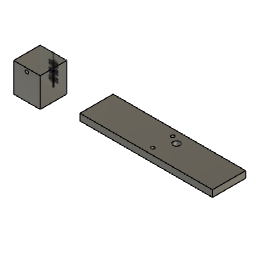
Phantom3 (Autodesk Fusion 360 design; units mm, degrees)
Autodesk Fusion 360 part; units mm, degrees
sketch "Sketch1" plane through (0, 0, 0) normal (0, 0, 1) x (1, 0, 0)
  line L0 (20, 20) -> (-20, 20)
  line L1 (-20, 20) -> (-20, -20)
  line L2 (-20, -20) -> (20, -20)
  line L3 (20, -20) -> (20, 20)
  line L4 (20, 20) -> (-20, -20) construction
  line L5 (-20, 20) -> (20, -20) construction
  line L6 (6, 20) -> (-6, 20)
  line L7 (-6, 20) -> (-6, -20)
  line L8 (-6, -20) -> (6, -20)
  line L9 (6, -20) -> (6, 20)
  line L10 (6, 20) -> (-6, -20) construction
  line L11 (-6, 20) -> (6, -20) construction
  line L12 (6, 6) -> (-6, 6)
  line L13 (-6, 6) -> (-6, -6)
  line L14 (-6, -6) -> (6, -6)
  line L15 (6, -6) -> (6, 6)
  line L16 (6, 6) -> (-6, -6) construction
  line L17 (-6, 6) -> (6, -6) construction
  dimension "d1" = 40
  dimension "d2" = 40
  dimension "d3" = 12
  dimension "d4" = 40
  dimension "d5" = 12
  constraint horizontal L0
  constraint perpendicular L0 L1
  constraint parallel L0 L2
  constraint parallel L1 L3
  constraint coincident L4 origin
  constraint coincident L5 origin
  constraint horizontal L6
  constraint perpendicular L6 L7
  constraint parallel L6 L8
  constraint parallel L7 L9
  constraint coincident L10 origin
  constraint coincident L11 origin
  constraint horizontal L12
  constraint perpendicular L12 L13
  constraint parallel L12 L14
  constraint parallel L13 L15
  constraint coincident L16 origin
  constraint coincident L17 origin
  measures "d1" distance of L1.end L2.end
  measures "d2" distance of L0.end L1.end
  measures "d3" distance of L7.end L8.end
  measures "d4" distance of L6.end L7.end
  measures "d5" distance of L12.end L13.end
extrude "Extrude1" add sketch "Sketch1" against normal blind 20 makes body 1
extrude "Extrude2" add sketch "Sketch1" along normal blind 4 contours L0 L2 L3 L9 L15 | L0 L1 L2 L7 L13 | L2 L7 L8 L9 L14 bodies 1
extrude "Extrude3" add sketch "Sketch1" along normal blind 4 contours L0 L6 L7 L9 L12 | L7 L9 L12 L13 L14 L15 bodies 1
extrude "Extrude4" add 1 faces at (-6.6667, 6.6667, 4) along direction (0, 0, 1) blind 20 on bodies 1 bodies 1
extrude "Extrude5" add sketch "Sketch1" along normal blind 4 separate body contours L0 L6 L7 L9 L12 | L7 L9 L12 L13 L14 L15 makes body 2
extrude "Extrude6" cut 1 faces at (2, 20, 1.3333) along direction (0, -1, 0) blind 26 on bodies 2 bodies 1 2
sketch "Sketch2" plane through (-20, 0, 0) normal (-1, 0, 0) x (0, -1, 0)
  line L0 (-20, 24) -> (-20, -20)
  line L1 (-20, -20) -> (20, -20)
  line L2 (20, -20) -> (20, 24)
  line L3 (20, 24) -> (-20, 24)
  line L4 (0, 24) -> (0, 19)
  circle A0 centre (0, 19) radius 2.5
  dimension "d18" = 5
  dimension "d19" = 5
  constraint midpoint L3 L4.start
  constraint perpendicular L3 L4
  constraint coincident L4.end A0.centre
  measures "d18" distance of L4.start L4.end
  measures "d19" diameter of A0
sketch "Sketch3" plane through (0, -20, 0) normal (0, -1, 0) x (1, 0, 0)
  line L0 (-20, 24) -> (-20, -20)
  line L1 (-20, -20) -> (20, -20)
  line L2 (20, -20) -> (20, 24)
  line L3 (20, 24) -> (-20, 24)
  line L4 (0, 24) -> (0, 19)
  circle A0 centre (0, 19) radius 2.5
  dimension "d20" = 5
  dimension "d21" = 5
  constraint midpoint L3 L4.start
  constraint perpendicular L3 L4
  constraint coincident L4.end A0.centre
  measures "d20" distance of L4.start L4.end
  measures "d21" diameter of A0
extrude "Extrude7" cut sketch "Sketch2" against normal blind 40 contours A0 bodies 1
extrude "Extrude8" cut sketch "Sketch3" against normal blind 40 contours A0 bodies 1
sketch "Sketch4" plane through (0, 20, 0) normal (0, 1, 0) x (-1, 0, 0)
  circle A0 centre (0, 19) radius 2.5
  line L0 (6, 4) -> (6, 0)
  line L1 (6, 0) -> (-6, 0)
  line L2 (-6, 0) -> (-6, 4)
  line L3 (-6, 4) -> (6, 4)
  line L4 (-20, 24) -> (-20, -20)
  line L5 (-20, -20) -> (20, -20)
  line L6 (20, -20) -> (20, 24)
  line L7 (20, 24) -> (-20, 24)
  line L8 (0, 24) -> (0, -20)
  line L9 (0, -20) -> (0, -10)
  line L10 (6, -12) -> (-6, -12)
  line L11 (-6, -12) -> (-6, -8)
  line L12 (-6, -8) -> (6, -8)
  line L13 (6, -8) -> (6, -12)
  line L14 (6, -12) -> (-6, -8) construction
  line L15 (-6, -12) -> (6, -8) construction
  line L16 (0, -20) -> (0, 10)
  line L17 (6, 8) -> (-6, 8)
  line L18 (-6, 8) -> (-6, 12)
  line L19 (-6, 12) -> (6, 12)
  line L20 (6, 12) -> (6, 8)
  line L21 (6, 8) -> (-6, 12) construction
  line L22 (-6, 8) -> (6, 12) construction
  line L23 (0, -20) -> (0, 0)
  line L24 (6, -2) -> (-6, -2)
  line L25 (-6, -2) -> (-6, 2)
  line L26 (-6, 2) -> (6, 2)
  line L27 (6, 2) -> (6, -2)
  line L28 (6, -2) -> (-6, 2) construction
  line L29 (-6, -2) -> (6, 2) construction
  point P0 (0, -10)
  point P1 (0, 10)
  dimension "d26" = 10
  dimension "d27" = 12
  dimension "d28" = 4
  dimension "d29" = 30
  dimension "d30" = 12
  dimension "d31" = 4
  dimension "d34" = 20
  dimension "d35" = 12
  dimension "d36" = 4
  constraint midpoint L7 L8.start
  constraint midpoint L5 L8.end
  constraint perpendicular L5 L9
  constraint horizontal L10
  constraint perpendicular L10 L11
  constraint parallel L10 L12
  constraint parallel L11 L13
  constraint coincident L14 P0
  constraint coincident L15 P0
  constraint coincident P0 L9.end
  constraint coincident L8 P1
  constraint horizontal L17
  constraint perpendicular L17 L18
  constraint parallel L17 L19
  constraint parallel L18 L20
  constraint coincident L21 P1
  constraint coincident L22 P1
  constraint coincident P1 L16.end
  constraint parallel L16 L23
  constraint horizontal L24
  constraint perpendicular L24 L25
  constraint parallel L24 L26
  constraint parallel L25 L27
  constraint coincident L28 L23.end
  constraint coincident L29 L23.end
  constraint coincident L23.end origin
  measures "d26" distance of L8.end P0
  measures "d27" distance of L11.end L12.end
  measures "d28" distance of L10.end L11.end
  measures "d29" distance of L8.end P1
  measures "d30" distance of L18.end L19.end
  measures "d31" distance of L17.end L18.end
  measures "d34" distance of L8.end L23.end
  measures "d35" distance of L25.end L26.end
  measures "d36" distance of L24.end L25.end
extrude "Extrude9" add sketch "Sketch4" against normal blind 12 contours L2 L3 L8 L16 L26 | L0 L3 L8 L16 L26 | L0 L1 L8 L16 L26 L27 | L1 L2 L8 L16 L25 L26 bodies 1 2
extrude "Extrude10" cut sketch "Sketch4" against normal blind 26 contours L8 L16 L17 L19 L20 | L8 L16 L17 L18 L19 | L8 L9 L10 L11 L12 L16 L23 | L8 L9 L10 L12 L13 L16 L23 | L0 L1 L8 L16 L26 L27 | L1 L2 L8 L16 L25 L26 | L1 L8 L16 L23 L24 L25 | L1 L8 L16 L23 L24 L27 bodies 1
extrude "Extrude11" cut sketch "Sketch4" against normal blind 40 contours L2 L3 L8 L16 L26 | L0 L3 L8 L16 L26 bodies 1
extrude "Extrude12" add sketch "Sketch4" against normal blind 40 contours L2 L3 L8 L16 L26 | L0 L3 L8 L16 L26 bodies 1
sketch "Sketch5" plane through (0, 0, 0) normal (0, 0, 1) x (1, 0, 0)
  line L0 (285, -25) -> (85, -25)
  line L1 (85, -25) -> (85, 25)
  line L2 (85, 25) -> (285, 25)
  line L3 (285, 25) -> (285, -25)
  line L4 (285, -25) -> (85, 25) construction
  line L5 (85, -25) -> (285, 25) construction
  circle A0 centre (185, 0) radius 15
  line L6 (185, 0) -> (185, 25)
  line L7 (185, 0) -> (185, -25)
  circle A1 centre (185, 15) radius 2.5
  circle A2 centre (185, -15) radius 2.5
  circle A3 centre (197.4932, 8.3018) radius 5
  point P0 (185, 0)
  dimension "d43" = 200
  dimension "d44" = 50
  dimension "d45" = 5
  dimension "d46" = 5
  dimension "d47" = 10
  constraint horizontal L0
  constraint perpendicular L0 L1
  constraint parallel L0 L2
  constraint parallel L1 L3
  constraint coincident L4 P0
  constraint coincident L5 P0
  constraint coincident P0 A0.centre
  constraint midpoint L2 L6.end
  constraint midpoint L0 L7.end
  constraint coincident A0 A1.centre
  constraint coincident L6 A1.centre
  constraint coincident L7 A2.centre
  constraint coincident A0 A2.centre
  constraint coincident A0 A3.centre
  measures "d43" distance of L1.end L2.end
  measures "d44" distance of L0.end L1.end
  measures "d45" diameter of A1
  measures "d46" diameter of A2
  measures "d47" diameter of A3
extrude "Extrude13" add sketch "Sketch5" along normal blind 10 separate body contours L0 L2 L3 A0 L6 L7 A1 A2 A3 | L0 L1 L2 A0 L6 L7 A1 A2 | A0 L6 L7 A1 A2 | A0 L6 L7 A1 A2 A3 makes body 3
